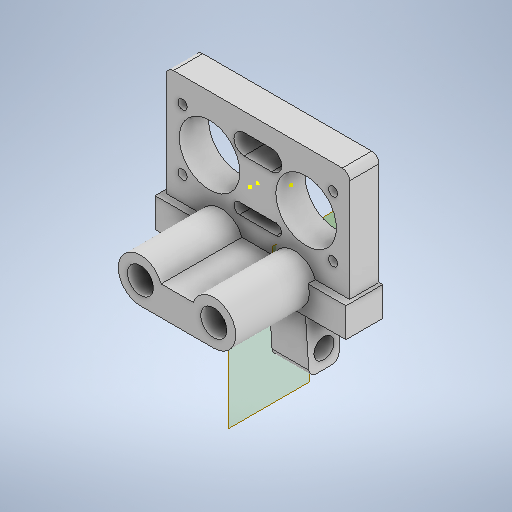
# Autodesk Inventor part: Czujnik_podstawa
Saved by Autodesk Inventor 2025.2 (Build 292293000, 293)
## iProperties
Created: 2025-11-25
Part Number: Czujnik_podstawa
Material: Ogólny
Document SubType Name: Modeling
Designer: juras
Density: 1 g/cm^3
Appearance: Domyślna
Author: juras
Autodesk Inventor part; units mm, degrees
ref_plane "YZ Plane" through (0, 0, 0) normal (1, 0, 0) x (0, 1, 0)
ref_plane "XZ Plane" through (0, 0, 0) normal (0, 1, 0) x (-1, 0, 0)
ref_plane "XY Plane" through (0, 0, 0) normal (0, 0, 1) x (1, 0, 0)
sketch "Szkic1" plane through (0, 0, 0) normal (0, 0, 1) x (1, 0, 0)
  line L0 (-25, -15) -> (25, -15)
  line L1 (25, -15) -> (25, 15)
  line L2 (25, 15) -> (-25, 15)
  line L3 (-25, 15) -> (-25, -15)
  line L4 (-25, -15) -> (25, 15) construction
  line L5 (25, -15) -> (-25, 15) construction
  point P0 (0, 0)
  dimension "d0" = 50
  dimension "d1" = 30
  constraints: 12 end point, 2 midpoint, 2 parallel, 1 horizontal, 1 perpendicular
  measures "d0" distance of L2.end L1.end
  measures "d1" distance of L1.end L0.end
extrude "Wyciągnięcie proste1" add sketch "Szkic1" along normal mid plane 8
sketch "Szkic8" plane through (0, 0, -4) normal (0, 0, -1) x (-1, 0, 0)
  line L0 (-20.5, -8.25) -> (20.5, -8.25)
  line L1 (20.5, -8.25) -> (20.5, 8.25)
  line L2 (20.5, 8.25) -> (-20.5, 8.25)
  line L3 (-20.5, 8.25) -> (-20.5, -8.25)
  line L4 (-20.5, -8.25) -> (20.5, 8.25) construction
  line L5 (20.5, -8.25) -> (-20.5, 8.25) construction
  point P0 (0, 0)
  dimension "d24" = 41
  dimension "d25" = 16.5
  constraints: 12 end point, 2 midpoint, 2 parallel, 1 horizontal, 1 perpendicular
  measures "d24" distance of L2.end L1.end
  measures "d25" distance of L0.end L1.end
hole "Otwór2" at (20.5, 8.25, -4) at (20.5, -8.25, -4) at (-20.5, 8.25, -4) at (-20.5, -8.25, -4) direction (0, 0, 1) diameter 2.5 depth 25 tip angle 118
sketch "Szkic9" plane through (0, 0, -4) normal (0, 0, -1) x (-1, 0, 0)
  line L0 (-22.5, -10) -> (22.5, -10)
  line L1 (22.5, -10) -> (22.5, 10)
  line L2 (22.5, 10) -> (-22.5, 10)
  line L3 (-22.5, 10) -> (-22.5, -10)
  line L4 (-22.5, -10) -> (22.5, 10) construction
  line L5 (22.5, -10) -> (-22.5, 10) construction
  circle A0 centre (-13.15, 0) radius 8.25
  line L6 (25, 15) -> (-25, 15) projected
  point P0 (0, 0)
  dimension "d33" = 45
  dimension "d34" = 20
  dimension "d35" = 16.5
  dimension "d36" = 9.35
  dimension "d38" = 10
  constraints: 12 end point, 2 midpoint, 2 parallel, 1 centre point, 1 horizontal, 1 perpendicular
  measures "d33" distance of L2.end L1.end
  measures "d34" distance of L1.end L0.end
  measures "d35" diameter of A0
  measures "d36" distance from line of A0.centre L3
  measures "d38" distance from line of A0.centre L2
extrude "Wyciągnięcie proste3" cut sketch "Szkic9" against normal blind 8 contours A0
mirror "Odbij1" about plane through (0, 0, 0) normal (1, 0, 0) of "Wyciągnięcie proste3"
sketch "Szkic10" plane through (0, 0, -4) normal (0, 0, -1) x (-1, 0, 0)
  line L0 (-22.5, -10) -> (22.5, -10)
  line L1 (22.5, -10) -> (22.5, 10)
  line L2 (22.5, 10) -> (-22.5, 10)
  line L3 (-22.5, 10) -> (-22.5, -10)
  line L4 (-22.5, -10) -> (22.5, 10) construction
  line L5 (22.5, -10) -> (-22.5, 10) construction
  line L6 (-3.75, 7.25) -> (3.75, 7.25) construction
  line L7 (-3.75, 10) -> (3.75, 10)
  line L8 (3.75, 4.5) -> (-3.75, 4.5)
  arc A0 (-3.75, 10) -> (-3.75, 4.5) centre (-3.75, 7.25) ccw
  arc A1 (3.75, 4.5) -> (3.75, 10) centre (3.75, 7.25) ccw
  line L9 (25, -15) -> (25, 15) projected
  line L10 (-5, -8.5) -> (5, -8.5) construction
  line L11 (-5, -10) -> (5, -10)
  line L12 (5, -7) -> (-5, -7)
  arc A2 (-5, -7) -> (-5, -10) centre (-5, -8.5) ccw
  arc A3 (5, -10) -> (5, -7) centre (5, -8.5) ccw
  point P0 (0, 0)
  point P1 (0, 7.25)
  point P2 (-6.5, 7.25)
  point P3 (6.5, 7.25)
  point P4 (0, -8.5)
  point P5 (-6.5, -8.5)
  point P6 (6.5, -8.5)
  point P7 (5, -10)
  point P8 (3.75, 10)
  dimension "d41" = 45
  dimension "d42" = 20
  dimension "d43" = 0
  dimension "d44" = 5.5
  dimension "d45" = 16
  dimension "d47" = 16
  dimension "d48" = 0
  dimension "d49" = 3
  dimension "d50" = 16
  dimension "d51" = 16
  constraints: 28 end point, 12 point on circle, 8 tangent, 4 centre point, 4 midpoint, 4 parallel, 3 horizontal, 1 perpendicular
  measures "d41" distance of L2.end L1.end
  measures "d42" distance of L1.end L0.end
  measures "d43" distance between parallel lines of L2 L7
  measures "d44" distance between parallel lines of L2 L8
  measures "d45" distance from line of L3 point (-6.5, 7.25)
  measures "d47" distance from line of L1 point (6.5, 7.25)
  measures "d48" distance between parallel lines of L0 L11
  measures "d49" distance between parallel lines of L0 L12
  measures "d50" distance from line of L3 point (-6.5, -8.5)
  measures "d51" distance from line of L1 point (6.5, -8.5)
extrude "Wyciągnięcie proste4" cut sketch "Szkic10" against normal blind 8 contours A2 L12 A3 L0 | L2 A1 L8 A0
fillet "Zaokrąglenie1" radius 2 2 edges at (25, 15, 0) (-25, 15, 0)
sketch "Szkic11" plane through (-25, -15, 4) normal (0, -1, 0) x (1, 0, 0)
  line L0 (51, -10) -> (-1, -10)
  line L1 (-1, -10) -> (-1, 2)
  line L2 (-1, 2) -> (51, 2)
  line L3 (51, 2) -> (51, -10)
  line L4 (51, -10) -> (-1, 2) construction
  line L5 (-1, -10) -> (51, 2) construction
  line L6 (50, -8) -> (0, -8) projected
  line L7 (0, -8) -> (0, 0) projected
  point P0 (25, -4)
  dimension "d55" = 2
  dimension "d57" = 52
  constraints: 12 end point, 2 midpoint, 2 parallel, 1 horizontal, 1 perpendicular
  measures "d55" distance between parallel lines of L6 L0
  measures "d57" distance of L1.end L2.end
extrude "Wyciągnięcie proste5" add sketch "Szkic11" along normal blind 8
ref_plane "Płaszczyzna konstrukcyjna3" through (5, -23, -6) normal (-1, 0, 0) x (0, 0, 1)
ref_plane "Płaszczyzna konstrukcyjna2" through (5, -23, -6) normal (-1, 0, 0) x (0, 0, 1)
ref_plane "Płaszczyzna konstrukcyjna1" through (5, -38, 6) normal (-1, 0, 0) x (0, 0, 1)
sketch "Szkic22" plane through (-26, -15, 6) normal (0, 0, 1) x (1, 0, 0)
  line L0 (8, -8) -> (44, -8)
  line L1 (44, -8) -> (44, 0)
  line L2 (44, 0) -> (8, 0)
  line L3 (8, 0) -> (8, -8)
  line L4 (8, -8) -> (44, 0) construction
  line L5 (44, -8) -> (8, 0) construction
  line L6 (0, 0) -> (0, -8) projected
  line L7 (52, 0) -> (52, -8) projected
  line L8 (52, 0) -> (0, 0) projected
  circle A0 centre (16, -2) radius 6
  circle A1 centre (16, -2) radius 3.55
  circle A2 centre (36, -2) radius 6
  line L9 (41, -8) -> (31, -8) projected
  circle A3 centre (36, -2) radius 3.55
  point P0 (26, 15)
  point P1 (26, -4)
  point P2 (21.6569, 0)
  point P3 (16, -8)
  point P4 (36, -8)
  point P5 (30.3431, 0)
  dimension "d109" = 8
  dimension "d110" = 8
  dimension "d111" = 8
  dimension "d112" = 0
  dimension "d113" = 6
  dimension "d114" = 12
  dimension "d115" = 8
  dimension "d116" = 7.1
  dimension "d123" = 8
  dimension "d124" = 12
  dimension "d125" = 7.1
  constraints: 12 end point, 4 centre point, 2 coincident, 2 midpoint, 2 parallel, 1 horizontal, 1 perpendicular, 1 tangent
  measures "d109" distance between parallel lines of L6 L3
  measures "d110" distance between parallel lines of L7 L1
  measures "d111" distance between parallel lines of L0 L2
  measures "d112" distance between parallel lines of L8 L2
  measures "d113" distance from line of L0 A0.centre
  measures "d114" diameter of A0
  measures "d115" distance from line of A0.centre L3
  measures "d116" diameter of A1
  measures "d123" distance from line of L1 A2.centre
  measures "d124" diameter of A2
  measures "d125" diameter of A3
extrude "Wyciągnięcie proste13" add sketch "Szkic22" along normal blind 20 contours L0 A0 L2 A2 | A2 L2 A3 | A2 L2 A3 | A0 L2 A1 | L2 A1 A0
sketch "Szkic23" plane through (-26, -15, 6) normal (0, 0, -1) x (-1, 0, 0)
  point P0 (-26, 15)
sketch "Szkic24" plane through (0, 0, 4) normal (0, 0, 1) x (1, 0, 0)
  point P0 (0, 0)
sketch "Szkic25" plane through (0, 0, 4) normal (0, 0, 1) x (1, 0, 0)
  arc A0 (-12.933, -15) -> (-7.067, -15) centre (-10, -17) ccw projected
  circle A1 centre (-10, -17) radius 6
  point P0 (0, 0)
  dimension "d128" = 12
  constraints: 1 centre point, 1 coincident
  measures "d128" diameter of A1
extrude "Wyciągnięcie proste14" add sketch "Szkic25" along normal blind 2
mirror "Odbij4" about plane through (0, 0, 0) normal (1, 0, 0) of "Wyciągnięcie proste14"
sketch "Szkic26" plane through (5, -23, -6) normal (-1, 0, 0) x (0, 0, 1)
  point P0 (6, 23)
sketch "Szkic27" plane through (-25, -23, 4) normal (0, -1, 0) x (1, 0, 0)
  line L0 (10, 2) -> (20, 2)
  line L1 (20, 2) -> (20, -8)
  line L2 (20, -8) -> (10, -8)
  line L3 (10, -8) -> (10, 2)
  line L4 (-1, 2) -> (-1, -10) projected
  line L5 (15, 2) -> (-1, 2) projected
  line L6 (-1, -10) -> (51, -10) projected
  point P0 (25, -4)
  dimension "d131" = 11
  dimension "d132" = 0
  dimension "d134" = 10
  dimension "d135" = 10
  constraints: 8 end point, 2 parallel, 1 horizontal, 1 perpendicular
  measures "d131" distance between parallel lines of L3 L4
  measures "d132" distance between parallel lines of L0 L5
  measures "d134" distance between parallel lines of L3 L1
  measures "d135" distance between parallel lines of L2 L0
extrude "Wyciągnięcie proste15" add sketch "Szkic27" along normal blind 15
sketch "Szkic28" plane through (-15, -23, -4) normal (-1, 0, 0) x (0, 0, 1)
  line L0 (0, -15) -> (10, -15) projected
  line L1 (10, -15) -> (9, -15)
  line L2 (10, 8) -> (10, 0) projected
  line L3 (9, -15) -> (10, 0)
  line L4 (10, 0) -> (10, -15)
  line L5 (0, -15) -> (1, -15)
  line L6 (1, -15) -> (0, 0)
  line L7 (0, 0) -> (0, -15)
  circle A0 centre (5, -10) radius 2.75
  point P0 (4, 23)
  dimension "d138" = 1
  dimension "d139" = 1
  dimension "d140" = 5
  dimension "d141" = 5
  dimension "d142" = 5.5
  constraints: 12 end point, 2 point on line, 1 centre point, 1 collinear, 1 perpendicular
  measures "d138" distance of L0.end L1.end
  measures "d139" distance of L0.start L5.end
  measures "d140" distance from line of A0.centre L0
  measures "d141" distance from line of A0.centre L7
  measures "d142" diameter of A0
extrude "Wyciągnięcie proste16" cut sketch "Szkic28" against normal blind 15
fillet "Zaokrąglenie4" radius 2 2 edges at (-10, -38, -3) (-10, -38, 5)
mirror "Odbij5" about plane through (0, 0, 0) normal (1, 0, 0) of "Wyciągnięcie proste16", "Wyciągnięcie proste15", "Zaokrąglenie4"
sketch "Szkic29" plane through (-25, -15, 4) normal (0, 1, 0) x (1, 0, 0)
  line L0 (-1, 10) -> (51, 10) projected
  line L1 (51, 10) -> (-1, 10)
  line L2 (-1, 10) -> (-1, 8)
  line L3 (-1, 8) -> (51, 8)
  line L4 (51, 8) -> (51, 10)
  point P0 (25, 4)
  dimension "d146" = 52
  dimension "d147" = 2
  constraints: 8 end point, 2 parallel, 1 horizontal, 1 perpendicular
  measures "d146" distance of L3.end L2.end
  measures "d147" distance of L2.end L1.end
extrude "Wyciągnięcie proste17" cut sketch "Szkic29" against normal blind 15
